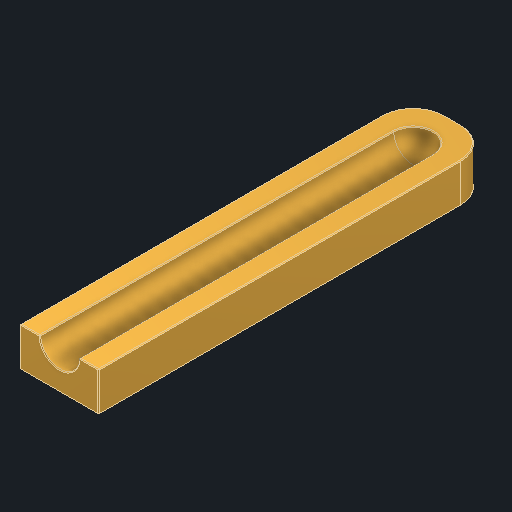
# Autodesk Inventor part: Ball Track
Saved by Autodesk Inventor 2027.1 (Build 311270010, 270A)
## iProperties
Created: 2025-09-16
Material: Brass, Soft Yellow
Document SubType Name: Modeling
Designer: SD
Density: 8.47 g/cm^3
Appearance: Brass - Satin
Mass: 135.26 g
Surface Area: 68.3211 cm^2
Volume: 15.9693 cm^3
Project: Automatic Tea Steeping mechanism
Part Number: Ball Track
Length: 100.000 mm
Thickness: 10.000 mm
Width: 20.000 mm
BOM-Mass: 0.13526
BOM-Area: 0.007
Procurement: Fabricate - 2nd round
Build Stage: 3
Preferred Material: C36000 Brass
Author: SD
Title: Ball Track
Autodesk Inventor part; units mm, degrees
ref_plane "YZ Plane" through (0, 0, 0) normal (1, 0, 0) x (0, 1, 0)
ref_plane "XZ Plane" through (0, 0, 0) normal (0, 1, 0) x (-1, 0, 0)
ref_plane "XY Plane" through (0, 0, 0) normal (0, 0, 1) x (1, 0, 0)
sketch "Sketch1" plane through (0, 0, 0) normal (0, 0, 1) x (1, 0, 0)
  line L0 (-10, 5) -> (10, 5)
  line L1 (10, 5) -> (10, -5)
  line L2 (10, -5) -> (-10, -5)
  line L3 (-10, -5) -> (-10, 5)
  line L4 (-10, 5) -> (10, -5) construction
  line L5 (10, 5) -> (-10, -5) construction
  point P0 (0, 0)
  constraints: 12 end point, 4 parallel, 2 midpoint, 1 horizontal, 1 perpendicular
extrude "Extrusion1" add sketch "Sketch1" along normal mid plane 100
sketch "Sketch8" plane through (0, 0, 50) normal (0, 0, 1) x (1, 0, 0)
  line L0 (-10, 5) -> (10, 5) projected
  line L1 (10, 5) -> (-10, 5) projected
  line L2 (-5, 5) -> (5, 5)
  line L3 (5, 5) -> (5, 0)
  line L4 (5, 0) -> (-5, 0)
  line L5 (-5, 0) -> (-5, 5)
  point P0 (0, 0)
  dimension "d32" = 5
  dimension "d33" = 10
  dimension "d34" = 5
  constraints: 8 end point, 2 parallel, 1 horizontal, 1 perpendicular, 1 point on line
  measures "d32" distance between parallel lines of L4 L0
  measures "d33" distance between parallel lines of L3 L5
  measures "d34" distance from line of point (0, 0) L5
extrude "Extrusion7" cut sketch "Sketch8" against normal blind 90
sketch "Sketch10" plane through (-10, 5, -50) normal (0, 1, 0) x (1, 0, 0)
  arc A0 (15, -10) -> (5, -10) centre (10, -10) ccw
  line L0 (5, -10) -> (15, -10) projected
  line L1 (10, -10) -> (10, -10) construction
  point P0 (10, -50)
  constraints: 2 end point, 2 point on circle, 1 centre point, 1 coincident, 1 midpoint, 1 vertical
extrude "Extrusion8" cut sketch "Sketch10" against normal blind 5
fillet "Fillet3" radius 5 3 edges at (0, 0, -45) (5, 0, 5) (-5, 0, 5)
fillet "Fillet4" radius 8 2 edges at (10, 0, -50) (-10, 0, -50)
chamfer "Chamfer2" distance 0.2 angle 45 28 edges at (10, 5, 4) (7.6569, 5, -47.6569) (0, 5, -50) (-7.6569, 5, -47.6569) (-10, 5, 4) (10, -5, 4) (7.6569, -5, -47.6569) (0, -5, -50) (-7.6569, -5, -47.6569) (-10, -5, 4) (10, 0, 50) (-10, 0, 50) (0, -5, 50) (-7.5, 5, 50) (-5, 5, 50) (7.5, 5, 50) (5, 5, 50) (-5, 5, 5) (-5, 5, -40) (-5, 4.9999, 5) (0, 5, -45) (5, 5, -40) (0, 4.9999, -45) (5, 5, 5) (5, 4.9999, 5) (-3.5356, 1.4644, 50) (0, 0, 50) (3.5356, 1.4644, 50)
sketch "Sketch11" plane through (-9.8, -5, 49.8) normal (0, -1, 0) x (1, 0, 0)
  line L0 (19.6, 0.2) -> (0, 0.2) projected
  line L1 (19.8, -91.8) -> (19.8, 0) projected
  point P0 (9.8, -59.8)
  point P1 (9.8, -59.8)
  dimension "d47" = 60
  dimension "d48" = 10
  constraints: 1 coincident
  measures "d47" distance from line of point (9.8, -59.8) L0
  measures "d48" distance from line of point (9.8, -59.8) L1
hole "Hole1" at (0, -5, -10) direction (0, 1, 0) diameter 2.459 depth 3.5 tip angle 118 thread size "M3x0.5" class "6H" standard "ISO Metric profile"
sketch "Sketch12" plane through (-10, -4.8, -42) normal (1, 0, 0) x (0, 0, -1)
  line L0 (-92, 9.6) -> (-92, 0) projected
  line L1 (-91.8, -0.2) -> (0, -0.2) projected
  point P0 (-42, 4.8)
  point P1 (-82, 3.8)
  point P2 (-72, 3.8)
  dimension "d49" = 10
  dimension "d50" = 10
  dimension "d51" = 4
  constraints: 1 horizontal alignment
  measures "d49" distance from line of point (-82, 3.8) L0
  measures "d50" distance of point (-72, 3.8) point (-82, 3.8)
  measures "d51" distance from line of point (-82, 3.8) L1
hole "Hole2" at (-10, -1, 40) at (-10, -1, 30) direction (1, 0, 0) diameter 2.459 depth 6 tip angle 118 thread size "M3x0.5" class "6H" standard "ISO Metric profile"
sketch "Sketch14" plane through (0, 0, -50) normal (0, 0, -1) x (-1, 0, 0)
  line L0 (-2, -5) -> (2, -5) projected
  point P0 (0, 0)
  point P1 (0, -1)
  dimension "d59" = 4
  constraints: 1 vertical alignment
  measures "d59" distance from line of point (0, -1) L0
hole "Hole3" at (0, -1, -50) direction (0, 0, 1) diameter 2.459 depth 6 tip angle 118 thread size "M3x0.5" class "6H" standard "ISO Metric profile"
body "Solid1"
